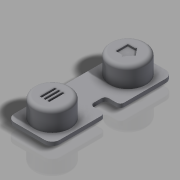
# Autodesk Inventor part: system-buttons
Saved by Autodesk Inventor 2019 (Build 230136000, 136)
## iProperties
Created: 2019-06-02
Part Number: system-buttons
Material: Generic
Document SubType Name: Modeling
Designer: jon
Density: 1 g/cm^3
Appearance: Default
Author: jon
Autodesk Inventor part; units mm, degrees
ref_plane "YZ Plane" through (0, 0, 0) normal (1, 0, 0) x (0, 1, 0)
ref_plane "XZ Plane" through (0, 0, 0) normal (0, 1, 0) x (-1, 0, 0)
ref_plane "XY Plane" through (0, 0, 0) normal (0, 0, 1) x (1, 0, 0)
sketch "Sketch1" plane through (0, 0, 0) normal (0, 1, 0) x (-1, 0, 0)
  line L0 (2, 8) -> (-2, 8)
  line L1 (-3, 7) -> (-3, 3)
  line L2 (-2, -8) -> (2, -8)
  line L3 (3, -7) -> (3, 7)
  circle A0 centre (0, 5) radius 2.4
  circle A1 centre (0, -5) radius 2.4
  arc A2 (3, 7) -> (2, 8) centre (2, 7) ccw
  arc A3 (-2, 8) -> (-3, 7) centre (-2, 7) ccw
  arc A4 (-3, -7) -> (-2, -8) centre (-2, -7) ccw
  arc A5 (2, -8) -> (3, -7) centre (2, -7) ccw
  line L4 (2, 2) -> (2, 2)
  line L5 (2, -2) -> (2, -2)
  line L6 (-2, 2) -> (-2, 2)
  line L7 (-2, -2) -> (-2, -2)
  line L8 (3, 3) -> (3, 7)
  line L9 (-3, 7) -> (-3, 1.5)
  line L10 (-2.5, -1) -> (-1.5, -1)
  line L11 (-1, -0.5) -> (-1, 0.5)
  line L12 (-1.5, 1) -> (-2.5, 1)
  line L13 (-3, -1.5) -> (-3, -7)
  arc A6 (-2.5, -1) -> (-3, -1.5) centre (-2.5, -1.5) ccw
  arc A7 (-3, 1.5) -> (-2.5, 1) centre (-2.5, 1.5) ccw
  arc A8 (-1.5, -1) -> (-1, -0.5) centre (-1.5, -0.5) ccw
  arc A9 (-1, 0.5) -> (-1.5, 1) centre (-1.5, 0.5) ccw
  point P0 (0, 0)
  point P1 (-3, -8)
  point P2 (-3, 8)
  point P3 (3, -8)
  point P4 (1, -2)
  point P5 (1, 2)
  point P6 (3, -2)
  point P7 (-3, 2)
  point P8 (-1, -2)
  point P9 (-3, -2)
  point P10 (-3, -1)
  point P11 (-1, 1)
  point P12 (-1, -1)
  point P13 (-3, 1)
  dimension "d0" = 6
  dimension "d1" = 16
  dimension "d2" = 4.8
  dimension "d3" = 4.8
  dimension "d5" = 3
  dimension "d6" = 1
  dimension "d7" = 2
  dimension "d8" = 4
  dimension "d9" = 2
  dimension "d70" = 2
  dimension "d71" = 2
  dimension "d72" = 0.5
  constraints: 28 end point, 26 point on line, 22 tangent, 16 point on circle, 10 centre point, 10 parallel, 6 equal radius, 4 horizontal, 4 perpendicular
  measures "d0" distance of point (3, -8) point (-3, -8)
  measures "d1" distance of point (-3, -8) point (-3, 8)
  measures "d2" diameter of A0
  measures "d3" diameter of A1
  measures "d5" distance from line of L3 point (0, 0)
  measures "d6" radius of A2
  measures "d7" distance of point (3, -2) point (1, -2)
  measures "d8" distance of point (1, -2) point (1, 2)
  measures "d9" distance of point (-1, -2) point (-3, -2)
  measures "d70" distance of point (-3, 1) point (-1, 1)
  measures "d71" distance of point (-1, 1) point (-1, -1)
  measures "d72" radius of A6
extrude "Extrusion1" add sketch "Sketch1" against normal blind 0.5 contours A2 L3 A5 L2 A4 L13 A6 L10 A8 L11 A9 L12 A7 L9 L1 A3 L0 | A0 | A1
extrude "Extrusion2" add sketch "Sketch1" along normal blind 2.65 contours A0 | A1
fillet "Fillet1" radius 0.5 2 edges at (2.4, 2.65, 5) (2.4, 2.65, -5)
sketch "Sketch2" plane through (0, -0.5, 0) normal (0, -1, 0) x (1, 0, 0)
  circle A0 centre (0, 5) radius 1.5
  circle A1 centre (0, -5) radius 1.5
  circle A2 centre (0, 5) radius 2
  circle A3 centre (0, -5) radius 2
  point P0 (0, 0)
  dimension "d18" = 3
  dimension "d19" = 3
  dimension "d22" = 4
  dimension "d23" = 4
  constraints: 4 centre point, 2 coincident
  measures "d18" diameter of A0
  measures "d19" diameter of A1
  measures "d22" diameter of A2
  measures "d23" diameter of A3
extrude "Extrusion3" cut sketch "Sketch2" against normal blind 2 contours A0 | A1
extrude "Extrusion4" add sketch "Sketch2" along normal blind 0.75
sketch "Sketch4" plane through (0, -0.5, 0) normal (0, -1, 0) x (1, 0, 0)
  line L0 (0.3, 6.75) -> (-0.3, 6.75)
  line L1 (-0.3, 6.75) -> (-0.3, 3.25)
  line L2 (-0.3, 3.25) -> (0.3, 3.25)
  line L3 (0.3, 3.25) -> (0.3, 6.75)
  line L4 (0.3, -3.25) -> (-0.3, -3.25)
  line L5 (-0.3, -3.25) -> (-0.3, -6.75)
  line L6 (-0.3, -6.75) -> (0.3, -6.75)
  line L7 (0.3, -6.75) -> (0.3, -3.25)
  circle A0 centre (0, 5) radius 1.5 projected
  circle A1 centre (0, -5) radius 1.5 projected
  circle A2 centre (0, 5) radius 0.3
  circle A3 centre (0, -5) radius 0.3
  point P0 (0, 0)
  dimension "d26" = 0.6
  dimension "d27" = 3.5
  dimension "d28" = 0.6
  dimension "d29" = 3.5
  dimension "d32" = 1.2
  dimension "d33" = 1.2
  dimension "d34" = 0.6
  dimension "d35" = 0.6
  constraints: 16 end point, 4 parallel, 2 centre point, 2 coincident, 2 horizontal, 2 perpendicular
  measures "d26" distance of L2.end L1.end
  measures "d27" distance of L1.end L0.end
  measures "d28" distance of L6.end L5.end
  measures "d29" distance of L5.end L4.end
  measures "d32" distance edge to line of A0 L3
  measures "d33" distance edge to line of A1 L7
  measures "d34" diameter of A2
  measures "d35" diameter of A3
extrude "Extrusion5" add sketch "Sketch4" against normal blind 2 and the other way blind 0.5 contours L3 A0 L1 L0 | L3 A2 L1 A0 | A2 | L3 A0 L1 A2 | A0 L3 L2 L1 | L7 A1 L5 L4 | L7 A3 L5 A1 | A3 | L7 A1 L5 A3 | A1 L7 L6 L5
extrude "Extrusion6" add sketch "Sketch4" along normal blind 0.75 contours A2 | A3
sketch "Sketch6" plane through (0, 2.65, 5) normal (0, 1, 0) x (1, 0, 0)
  line L0 (0.625, 1) -> (0.375, 1)
  line L1 (0.375, 1) -> (0.375, -1)
  line L2 (0.375, -1) -> (0.625, -1)
  line L3 (0.625, -1) -> (0.625, 1)
  line L4 (0.125, -1) -> (0.125, 1)
  line L5 (0.125, 1) -> (-0.125, 1)
  line L6 (-0.125, 1) -> (-0.125, -1)
  line L7 (-0.125, -1) -> (0.125, -1)
  line L8 (-0.375, -1) -> (-0.375, 1)
  line L9 (-0.375, 1) -> (-0.625, 1)
  line L10 (-0.625, 1) -> (-0.625, -1)
  line L11 (-0.625, -1) -> (-0.375, -1)
  point P0 (0, 5)
  point P1 (0, 0)
  dimension "d47" = 0.25
  dimension "d48" = 2
  dimension "d50" = 1
  dimension "d54" = 0.5
  dimension "d59" = 0.625
  constraints: 24 end point, 2 horizontal, 2 parallel, 1 collinear, 1 perpendicular, 16 other
  measures "d47" distance of L2.end L1.end
  measures "d48" distance of L1.end L0.end
  measures "d50" distance from line of L2 point (0, 0)
  measures "d54" distance of L2.end L4.start
  measures "d59" distance from line of point (0, 0) L3
sketch "Sketch5" plane through (0, 2.65, -5) normal (0, 1, 0) x (1, 0, 0)
  line L0 (-0.8, 0.8) -> (0.2, 0.8)
  line L1 (0.2, -0.8) -> (-0.8, -0.8)
  line L2 (-0.8, -0.8) -> (-0.8, 0.8)
  line L3 (0.2, 0.8) -> (0.2, 1.0087)
  line L4 (0.2, 1.0087) -> (1.0464, 0)
  line L5 (1.0464, 0) -> (0.2, -1.0087)
  line L6 (0.2, -1.0087) -> (0.2, -0.8)
  point P0 (0, -5)
  point P1 (0, 0)
  point P2 (0, 0)
  dimension "d40" = 40
  dimension "d41" = 100
  dimension "d43" = 1.6
  dimension "d44" = 1
  dimension "d62" = 0.8
  dimension "d69" = 0.8
  constraints: 14 end point, 1 coincident, 1 horizontal, 1 parallel, 1 perpendicular, 1 point on line, 1 vertical, 1 other
  measures "d40" angle of L3 L4
  measures "d41" angle of L4 L5
  measures "d43" distance between parallel lines of L1 L0
  measures "d44" distance between parallel lines of L2 L6
  measures "d62" distance from line of L1 point (0, 0)
  measures "d69" distance from line of L2 point (0, 0)
extrude "Extrusion7" cut sketch "Sketch5" against normal blind 0.25
extrude "Extrusion8" cut sketch "Sketch6" against normal blind 0.25
fillet "Fillet6" radius 0.05 7 edges at (-0.8, 2.525, -5.8) (0.2, 2.525, -5.8) (0.2, 2.525, -6.0087) (1.0464, 2.525, -5) (0.2, 2.525, -3.9913) (0.2, 2.525, -4.2) (-0.8, 2.525, -4.2)
fillet "Fillet9" radius 0.05 12 edges at (0.625, 2.525, 6) (0.125, 2.525, 6) (-0.375, 2.525, 6) (0.625, 2.525, 4) (0.125, 2.525, 4) (-0.375, 2.525, 4) (0.375, 2.525, 4) (-0.125, 2.525, 4) (-0.625, 2.525, 4) (0.375, 2.525, 6) (-0.125, 2.525, 6) (-0.625, 2.525, 6)
body "Solid1"
